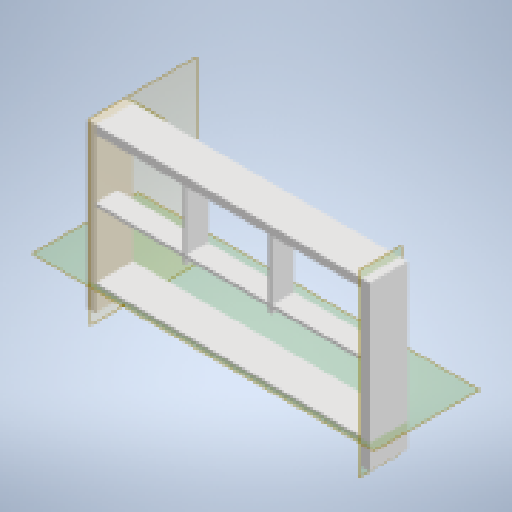
# Autodesk Inventor part: case
Saved by Autodesk Inventor 2024.3 (Build 283343000, 343)
## iProperties
Created: 2025-06-10
Part Number: case
Material: Generic
Document SubType Name: Modeling
Designer: megha
Density: 1 g/cm^3
Appearance: Default
Author: megha
Autodesk Inventor part; units mm, degrees
ref_plane "YZ Plane" through (0, 0, 0) normal (1, 0, 0) x (0, 1, 0)
ref_plane "XZ Plane" through (0, 0, 0) normal (0, 1, 0) x (-1, 0, 0)
ref_plane "XY Plane" through (0, 0, 0) normal (0, 0, 1) x (1, 0, 0)
ref_plane "boardTop(tolerance)" through (29.1257, 19.6924, 40.7272) normal (0, -1, 0) x (1, 0, 0)
sketch "Sketch3" plane through (29.1257, 19.6924, 40.7272) normal (0, -1, 0) x (1, 0, 0)
  line L0 (-2, 1.51) -> (-2, 0)
  line L1 (158.35, 0) -> (158.35, 1.51)
  line L2 (-8, 18.0177) -> (-8, -5)
  line L3 (164.35, 18.0177) -> (164.35, -5)
  line L4 (164.35, 18.0177) -> (-8, 18.0177)
  line L5 (-8, -5) -> (164.35, -5)
  point P0 (-29.1257, -40.7272)
  point P1 (158.35, 0.755)
  dimension "d12" = 6
  dimension "d13" = 6
  constraints: 12 end point, 1 horizontal, 1 midpoint, 1 parallel, 1 vertical, 2 other
  measures "d12" distance between parallel lines of L2 L0
  measures "d13" distance from line of point (158.35, 0.755) L3
extrude "Extrusion3" add sketch "Sketch3" against normal blind 5
ref_plane "boardBottom(tolerance)" through (185.4757, -59.8376, 42.2372) normal (0, -1, 0) x (-1, 0, 0)
sketch "Sketch4" plane through (29.1257, 19.6924, 40.7272) normal (0, -1, 0) x (1, 0, 0)
  line L0 (-2, 1.51) -> (-2, 0)
  line L1 (158.35, 1.51) -> (158.35, 0)
  line L2 (-8, 18.0177) -> (-8, -5) projected
  line L3 (-8, -5) -> (164.35, -5) projected
  line L4 (164.35, -5) -> (164.35, 18.0177) projected
  line L5 (164.35, 18.0177) -> (-8, 18.0177) projected
  line L6 (159.35, -5) -> (159.35, 18.0177)
  line L7 (-8, 18.0177) -> (164.35, 18.0177) projected
  line L8 (-3, -5) -> (-3, 18.0177)
  point P0 (-29.1257, -40.7272)
  point P1 (158.35, 0.755)
  point P2 (-2, 0.755)
  point P3 (-3, 18.0177)
  dimension "d17" = 1
  dimension "d18" = 1
  constraints: 8 end point, 4 point on line, 2 midpoint, 2 perpendicular, 2 vertical, 4 other
  measures "d17" distance from line of point (158.35, 0.755) L6
  measures "d18" distance from line of point (-2, 0.755) L8
extrude "Extrusion4" add sketch "Sketch4" along normal blind 94.5274 contours L5 L8 L3 L2 | L5 L4 L3 L6
ref_plane "boardRight(tolerance)" through (188.4757, 19.6924, 35.7272) normal (-1, 0, 0) x (0, -1, 0)
sketch "Sketch5" plane through (188.4757, -74.835, 35.7272) normal (-1, 0, 0) x (0, 0, 1)
  line L0 (5, 15.9974) -> (6.51, 15.9974) projected
  line L1 (0, 94.5274) -> (23.0177, 94.5274) projected
  line L2 (0, 94.5274) -> (0, 0) projected
  line L3 (23.0177, 0) -> (0, 0) projected
  line L4 (23.0177, 94.5274) -> (23.0177, 0) projected
  line L5 (0, 94.5274) -> (0, 0) projected
  line L6 (0, 15.9974) -> (23.0177, 15.9974)
  line L7 (23.0177, 15.9974) -> (23.0177, 12.9974)
  line L8 (23.0177, 12.9974) -> (0, 12.9974)
  line L9 (0, 12.9974) -> (0, 15.9974)
  point P0 (-35.7272, 74.835)
  point P1 (0, 12.9974)
  point P2 (6.51, 15.9974)
  dimension "d21" = 3
  constraints: 8 end point, 2 horizontal, 2 parallel, 2 point on line, 1 perpendicular
  measures "d21" distance of L6.end L7.end
ref_plane "boardLeft(tolerance)" through (26.1257, 19.6924, 58.7449) normal (1, 0, 0) x (0, -1, 0)
extrude "Extrusion5" add sketch "Sketch5" along normal up to surface (162.35 mm away) contours L0 L6 L4 L8 L2
sketch "Sketch6" plane through (29.1257, 19.6924, 40.7272) normal (0, -1, 0) x (1, 0, 0)
  line L0 (48.3131, 6.295) -> (48.54, 4.395) projected
  line L1 (54.3069, 2.495) -> (54.08, 4.395) projected
  line L2 (99.8531, 6.295) -> (100.08, 4.395) projected
  line L3 (107.5969, 2.495) -> (107.37, 4.395) projected
  line L4 (-3, 18.0177) -> (-3, -5) projected
  line L5 (-3, -5) -> (159.35, -5) projected
  line L6 (159.35, -5) -> (159.35, 18.0177) projected
  line L7 (159.35, 18.0177) -> (-3, 18.0177) projected
  line L8 (0, 1.51) -> (156.35, 1.51) projected
  line L9 (102.725, 1.51) -> (104.725, 1.51)
  line L10 (104.725, 1.51) -> (104.725, 18.0177)
  line L11 (104.725, 18.0177) -> (102.725, 18.0177)
  line L12 (102.725, 18.0177) -> (102.725, 1.51)
  line L13 (159.35, 18.0177) -> (-3, 18.0177) projected
  line L14 (50.31, 1.51) -> (52.31, 1.51)
  line L15 (52.31, 1.51) -> (52.31, 18.0177)
  line L16 (52.31, 18.0177) -> (50.31, 18.0177)
  line L17 (50.31, 18.0177) -> (50.31, 1.51)
  line L18 (48.4266, 5.345) -> (50.31, 5.345) construction
  line L19 (54.1934, 3.445) -> (52.31, 3.445) construction
  line L20 (99.9666, 5.345) -> (102.725, 5.345) construction
  line L21 (107.4834, 3.445) -> (104.725, 3.445) construction
  point P0 (-29.1257, -40.7272)
  point P1 (124.6421, 15.795)
  dimension "d31" = 2
  dimension "d32" = 2
  constraints: 24 end point, 8 point on line, 6 parallel, 6 perpendicular, 4 midpoint, 2 horizontal, 1 other
  measures "d31" distance between parallel lines of L17 L15
  measures "d32" distance between parallel lines of L10 L12
extrude "Extrusion6" add sketch "Sketch6" along normal blind 41.275 contours L7 L15 L8 L17 | L7 L10 L8 L12
sketch "Sketch7" plane through (133.8507, 19.6924, 42.2372) normal (0, 0, -1) x (-1, 0, 0)
  line L0 (2, 0) -> (2, -41.275) projected
  line L1 (0, 0) -> (0, -41.275) projected
  line L2 (2, -41.275) -> (0, -41.275) projected
  line L3 (54.415, 0) -> (54.415, -41.275) projected
  line L4 (52.415, 0) -> (52.415, -41.275) projected
  line L5 (54.415, -41.275) -> (52.415, -41.275) projected
  line L6 (0, 0) -> (2, 0)
  line L7 (54.415, 0) -> (52.415, 0)
  point P0 (133.8507, -19.6924)
  constraints: 4 end point, 1 collinear, 1 horizontal
extrude "Extrusion7" cut sketch "Sketch7" against normal blind 3
sketch "Sketch9" plane through (188.4757, 19.6924, 35.7272) normal (-1, 0, 0) x (0, 0, 1)
  line L0 (23.0177, 0) -> (23.0177, -41.275) projected
  line L1 (23.0177, -41.275) -> (9.51, -41.275) projected
  line L2 (9.51, 0) -> (9.51, -41.275) projected
  line L3 (9.51, -38.275) -> (23.0177, -38.275)
  line L4 (23.0177, 0) -> (23.0177, -78.53) projected
  line L5 (9.51, -36.275) -> (23.0177, -36.275)
  point P0 (-35.7272, -19.6924)
  point P1 (23.0177, -36.275)
  point P2 (23.0177, -38.275)
  dimension "d35" = 3
  dimension "d37" = 2
  constraints: 4 end point, 4 point on line, 2 horizontal
  measures "d35" distance between parallel lines of L1 L3
  measures "d37" distance between parallel lines of L3 L5
extrude "Extrusion8" add sketch "Sketch9" along normal up to surface (162.35 mm away) contours L0 L3 L2 L5
body "Solid2"
